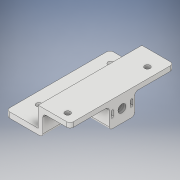
# Autodesk Inventor part: Dual Camera Mount
Saved by Autodesk Inventor 2019 (Build 230136000, 136)
## iProperties
Created: 2020-02-21
Part Number: Dual Camera Mount
Material: Generic
Document SubType Name: Modeling
Designer: close
Density: 1 g/cm^3
Appearance: Smooth - White
Author: close
Autodesk Inventor part; units mm, degrees
ref_plane "YZ Plane" through (0, 0, 0) normal (1, 0, 0) x (0, 1, 0)
ref_plane "XZ Plane" through (0, 0, 0) normal (0, 1, 0) x (-1, 0, 0)
ref_plane "XY Plane" through (0, 0, 0) normal (0, 0, 1) x (1, 0, 0)
sketch "Sketch1" plane through (0, 0, 0) normal (0, 1, 0) x (-1, 0, 0)
  line L0 (0, 0) -> (40, 0)
  line L1 (40, 0) -> (40, -65)
  line L2 (40, -65) -> (0, -65)
  line L3 (0, -65) -> (0, 0)
  dimension "d0" = 40
  dimension "d1" = 65
  constraints: 8 end point, 2 parallel, 1 horizontal, 1 perpendicular
  measures "d0" distance between parallel lines of L3 L1
  measures "d1" distance between parallel lines of L2 L0
extrude "Extrusion1" add sketch "Sketch1" along normal blind 16
sketch "Sketch2" plane through (-40, 0, 0) normal (0, 0, 1) x (1, 0, 0)
  line L0 (0, 16) -> (40, 16) projected
  line L1 (0, 16) -> (20, 16)
  line L2 (20, 16) -> (20, 3.5)
  line L3 (20, 3.5) -> (0, 3.5)
  line L4 (0, 3.5) -> (0, 16)
  line L5 (40, 0) -> (0, 0) projected
  dimension "d4" = 20
  dimension "d5" = 3.5
  constraints: 8 end point, 2 parallel, 1 horizontal, 1 perpendicular
  measures "d4" distance between parallel lines of L4 L2
  measures "d5" distance between parallel lines of L5 L3
extrude "Extrusion2" cut sketch "Sketch2" against normal through all
sketch "Sketch3" plane through (0, 0, 0) normal (0, -1, 0) x (1, 0, 0)
  line L0 (-32.5, -58) -> (-32.5, -13) construction
  line L1 (-6.5, -55) -> (-6.5, -5) construction
  line L2 (-40, -65) -> (0, -65) construction
  line L3 (0, 0) -> (-40, 0) construction
  line L4 (0, -65) -> (0, 0) construction
  line L5 (-40, 0) -> (-40, -65) construction
  dimension "d8" = 45
  dimension "d9" = 50
  dimension "d10" = 7
  dimension "d11" = 5
  dimension "d12" = 6.5
  dimension "d13" = 7.5
  constraints: 4 end point, 2 vertical
  measures "d8" distance of L0.start L0.end
  measures "d9" distance of L1.start L1.end
  measures "d10" distance from line of L2 L0.start
  measures "d11" distance from line of L3 L1.end
  measures "d12" distance between parallel lines of L4 L1
  measures "d13" distance from line of L5 L0.end
hole "Hole1" at (-32.5, 0, -58) at (-32.5, 0, -13) at (-6.5, 0, -55) at (-6.5, 0, -5) direction (0, 1, 0) diameter 3.4 end through all clearance for "Flat Head Machine Screw" size "M3" standard "Ansi Metric M Profile"
sketch "Sketch4" plane through (0, 0, 0) normal (1, 0, 0) x (0, 0, -1)
  line L0 (38.5, 6.5) -> (38.5, 9.5) construction
  line L1 (39.25, 6.5) -> (39.25, 9.5)
  line L2 (37.75, 9.5) -> (37.75, 6.5)
  arc A0 (37.75, 6.5) -> (39.25, 6.5) centre (38.5, 6.5) ccw
  arc A1 (39.25, 9.5) -> (37.75, 9.5) centre (38.5, 9.5) ccw
  line L3 (26.5, 6.5) -> (26.5, 9.5) construction
  line L4 (27.25, 6.5) -> (27.25, 9.5)
  line L5 (25.75, 9.5) -> (25.75, 6.5)
  arc A2 (25.75, 6.5) -> (27.25, 6.5) centre (26.5, 6.5) ccw
  arc A3 (27.25, 9.5) -> (25.75, 9.5) centre (26.5, 9.5) ccw
  line L6 (0, 0) -> (0, 16) construction
  line L7 (65, 0) -> (65, 16) construction
  line L8 (38.5, 8) -> (26.5, 8) construction
  line L9 (65, 0) -> (0, 0) construction
  line L10 (0, 16) -> (65, 16) construction
  line L11 (65, 0) -> (40.5, 0)
  line L12 (40.5, 0) -> (40.5, 13)
  line L13 (40.5, 13) -> (65, 13)
  line L14 (65, 13) -> (65, 0)
  line L15 (24.5, 0) -> (0, 0)
  line L16 (0, 0) -> (0, 13)
  line L17 (0, 13) -> (24.5, 13)
  line L18 (24.5, 13) -> (24.5, 0)
  point P0 (32.5, 8)
  dimension "d21" = 12
  dimension "d22" = 6
  dimension "d23" = 65
  dimension "d24" = 32.5
  dimension "d25" = 3
  dimension "d26" = 3
  dimension "d27" = 0.75
  dimension "d28" = 0.75
  dimension "d29" = 0
  dimension "d30" = 16
  dimension "d31" = 8
  dimension "d32" = 3
  dimension "d33" = 3
  dimension "d34" = 16
  dimension "d35" = 8
  constraints: 34 end point, 8 parallel, 8 point on circle, 8 tangent, 4 centre point, 2 horizontal, 2 midpoint, 2 perpendicular, 2 point on line, 1 vertical
  measures "d21" distance between parallel lines of L3 L0
  measures "d22" distance from line of L0 point (32.5, 8)
  measures "d23" distance between parallel lines of L6 L7
  measures "d24" distance from line of L7 point (32.5, 8)
  measures "d25" distance of L0.start L0.end
  measures "d26" distance of L3.start L3.end
  measures "d27" radius of A2
  measures "d28" radius of A0
  measures "d29" distance from line of L8 point (32.5, 8)
  measures "d30" distance between parallel lines of L9 L10
  measures "d31" distance from line of L10 point (32.5, 8)
  measures "d32" distance between parallel lines of L10 L13
  measures "d33" distance between parallel lines of L10 L17
  measures "d34" distance between parallel lines of L12 L18
  measures "d35" distance from line of point (32.5, 8) L18
extrude "Extrusion3" cut sketch "Sketch4" against normal blind 2 contours A0 L2 A1 L1 | A2 L5 A3 L4
extrude "Extrusion4" cut sketch "Sketch4" against normal blind 17 contours L11 L12 L13 L14 | L15 L16 L17 L18
fillet "Fillet1" radius 2 14 edges at (-8.5, 0, -40.5) (-8.5, 0, -24.5) (-40, 1.75, -65) (-40, 1.75, 0) (0, 14.5, 0) (0, 14.5, -65) (-17, 0, -52.75) (-17, 0, -12.25) (-17, 6.5, -40.5) (-17, 6.5, -24.5) (-17, 13, -52.75) (-8.5, 13, -40.5) (-17, 13, -12.25) (-8.5, 13, -24.5)
hole "Hole2" at (0, 8, -32.5) direction (-1, 0, 0) diameter 4.978 depth 10 tip angle 118 thread size "1/4-20 UNC" class "2B" standard "ANSI Unified Screw Threads"
equation "\"d22\" = 0.5 * d21"
equation "\"d24\" = 0.5 * d23"
equation "\"d26\" = d25"
equation "\"d28\" = d27"
equation "\"d31\" = 0.5 * d30"
equation "\"d35\" = 0.5 * d34"
body "Solid1"
